Autodesk Inventor part; units mm, degrees
(part 2 of 2)
  line L144 (10.3485, -202.6701) -> (10.3485, -202.018)
  spline S172 degree 2 poles (10.3485, -202.018) (10.5375, -201.9254) (11.2155, -201.7439) (11.5193, -201.7439) knots 0 0 0 1 2 2 2
  spline S173 degree 2 poles (11.5193, -201.7439) (12.1603, -201.7439) (12.8828, -202.4219) (12.8828, -202.9999) knots 0 0 0 1 2 2 2
  spline S174 degree 2 poles (12.8828, -202.9999) (12.8828, -203.2703) (12.7568, -203.7224) (12.6456, -203.915) knots 0 0 0 1 2 2 2
  spline S175 degree 2 poles (12.6456, -203.915) (12.5345, -204.1151) (12.2122, -204.5078) (12.0343, -204.6968) knots 0 0 0 1 2 2 2
  spline S176 degree 2 poles (12.0343, -204.6968) (11.7453, -205.0117) (11.0377, -205.686) (10.8265, -205.8824) knots 0 0 0 1 2 2 2
  line L145 (10.8265, -205.8824) -> (13.0717, -205.8824)
  line L146 (13.0717, -205.8824) -> (13.0717, -206.4122)
  spline S177 degree 2 poles (14.9168, -202.2737) (14.7501, -202.2737) (14.4203, -202.3552) (14.261, -202.4182) knots 0 0 0 1 2 2 2
  spline S178 degree 2 poles (14.261, -202.4182) (14.1128, -202.4812) (13.8942, -202.6146) (13.809, -202.6738) knots 0 0 0 1 2 2 2
  line L147 (13.809, -202.6738) -> (13.772, -202.6738)
  line L148 (13.772, -202.6738) -> (13.772, -202.0255)
  spline S179 degree 2 poles (13.772, -202.0255) (13.972, -201.918) (14.6575, -201.7439) (14.965, -201.7439) knots 0 0 0 1 2 2 2
  spline S180 degree 2 poles (14.965, -201.7439) (15.2762, -201.7439) (15.7393, -201.8698) (15.9283, -202.0032) knots 0 0 0 1 2 2 2
  spline S181 degree 2 poles (15.9283, -202.0032) (16.1284, -202.1477) (16.3358, -202.5664) (16.3358, -202.848) knots 0 0 0 1 2 2 2
  spline S182 degree 2 poles (16.3358, -202.848) (16.3358, -203.2259) (15.8394, -203.7965) (15.4911, -203.8706) knots 0 0 0 1 2 2 2
  line L149 (15.4911, -203.8706) -> (15.4911, -203.915)
  spline S183 degree 2 poles (15.4911, -203.915) (15.6356, -203.9447) (15.9653, -204.078) (16.1061, -204.2114) knots 0 0 0 1 2 2 2
  spline S184 degree 2 poles (16.1061, -204.2114) (16.2469, -204.3411) (16.4248, -204.7561) (16.4248, -205.0562) knots 0 0 0 1 2 2 2
  spline S185 degree 2 poles (16.4248, -205.0562) (16.4248, -205.3637) (16.2136, -205.8861) (16.0209, -206.0862) knots 0 0 0 1 2 2 2
  spline S186 degree 2 poles (16.0209, -206.0862) (15.8208, -206.2936) (15.254, -206.5085) (14.8946, -206.5085) knots 0 0 0 1 2 2 2
  spline S187 degree 2 poles (14.8946, -206.5085) (14.55, -206.5085) (13.8757, -206.3418) (13.646, -206.227) knots 0 0 0 1 2 2 2
  line L150 (13.646, -206.227) -> (13.646, -205.5786)
  line L151 (13.646, -205.5786) -> (13.6905, -205.5786)
  spline S188 degree 2 poles (13.6905, -205.5786) (13.8831, -205.7194) (14.5352, -205.9787) (14.8575, -205.9787) knots 0 0 0 1 2 2 2
  spline S189 degree 2 poles (14.8575, -205.9787) (15.0465, -205.9787) (15.4244, -205.8602) (15.5504, -205.7231) knots 0 0 0 1 2 2 2
  spline S190 degree 2 poles (15.5504, -205.7231) (15.6726, -205.586) (15.8023, -205.2599) (15.8023, -205.0117) knots 0 0 0 1 2 2 2
  spline S191 degree 2 poles (15.8023, -205.0117) (15.8023, -204.7635) (15.6578, -204.4411) (15.5282, -204.3485) knots 0 0 0 1 2 2 2
  spline S192 degree 2 poles (15.5282, -204.3485) (15.3985, -204.2559) (15.0465, -204.1855) (14.839, -204.1855) knots 0 0 0 1 2 2 2
  line L152 (14.839, -204.1855) -> (14.5797, -204.1855)
  line L153 (14.5797, -204.1855) -> (14.5797, -203.6779)
  line L154 (14.5797, -203.6779) -> (14.7834, -203.6779)
  spline S193 degree 2 poles (14.7834, -203.6779) (15.1947, -203.6779) (15.7134, -203.2852) (15.7134, -202.911) knots 0 0 0 1 2 2 2
  spline S194 degree 2 poles (15.7134, -202.911) (15.7134, -202.7368) (15.58, -202.4886) (15.4726, -202.4145) knots 0 0 0 1 2 2 2
  spline S195 degree 2 poles (15.4726, -202.4145) (15.3577, -202.3367) (15.0761, -202.2737) (14.9168, -202.2737) knots 0 0 0 1 2 2 2
  line L155 (19.0146, -201.6364) -> (17.2251, -207.4052)
  line L156 (17.2251, -207.4052) -> (16.7063, -207.4052)
  line L157 (16.7063, -207.4052) -> (18.4885, -201.6364)
  line L158 (18.4885, -201.6364) -> (19.0146, -201.6364)
  line L159 (22.338, -206.4122) -> (19.5185, -206.4122)
  line L160 (19.5185, -206.4122) -> (19.5185, -205.7638)
  spline S196 degree 2 poles (19.5185, -205.7638) (19.8223, -205.4785) (20.3632, -204.9487) (20.6226, -204.6634) knots 0 0 0 1 2 2 2
  spline S197 degree 2 poles (20.6226, -204.6634) (21.145, -204.0892) (21.5266, -203.4) (21.5266, -203.0332) knots 0 0 0 1 2 2 2
  spline S198 degree 2 poles (21.5266, -203.0332) (21.5266, -202.8406) (21.408, -202.5516) (21.3006, -202.4589) knots 0 0 0 1 2 2 2
  spline S199 degree 2 poles (21.3006, -202.4589) (21.1931, -202.3663) (20.9116, -202.2737) (20.7411, -202.2737) knots 0 0 0 1 2 2 2
  spline S200 degree 2 poles (20.7411, -202.2737) (20.5781, -202.2737) (20.2446, -202.3552) (20.0927, -202.4182) knots 0 0 0 1 2 2 2
  spline S201 degree 2 poles (20.0927, -202.4182) (19.9631, -202.4701) (19.7222, -202.6183) (19.6481, -202.6701) knots 0 0 0 1 2 2 2
  line L161 (19.6481, -202.6701) -> (19.6148, -202.6701)
  line L162 (19.6148, -202.6701) -> (19.6148, -202.018)
  spline S202 degree 2 poles (19.6148, -202.018) (19.8037, -201.9254) (20.4818, -201.7439) (20.7856, -201.7439) knots 0 0 0 1 2 2 2
  spline S203 degree 2 poles (20.7856, -201.7439) (21.4266, -201.7439) (22.149, -202.4219) (22.149, -202.9999) knots 0 0 0 1 2 2 2
  spline S204 degree 2 poles (22.149, -202.9999) (22.149, -203.2703) (22.0231, -203.7224) (21.9119, -203.915) knots 0 0 0 1 2 2 2
  spline S205 degree 2 poles (21.9119, -203.915) (21.8008, -204.1151) (21.4784, -204.5078) (21.3006, -204.6968) knots 0 0 0 1 2 2 2
  spline S206 degree 2 poles (21.3006, -204.6968) (21.0116, -205.0117) (20.3039, -205.686) (20.0927, -205.8824) knots 0 0 0 1 2 2 2
  line L163 (20.0927, -205.8824) -> (22.338, -205.8824)
  line L164 (22.338, -205.8824) -> (22.338, -206.4122)
  spline S207 degree 2 poles (25.7948, -204.1262) (25.7948, -205.3563) (25.0797, -206.5085) (24.335, -206.5085) knots 0 0 0 1 2 2 2
  spline S208 degree 2 poles (24.335, -206.5085) (23.5792, -206.5085) (22.8715, -205.334) (22.8715, -204.1299) knots 0 0 0 1 2 2 2
  spline S209 degree 2 poles (22.8715, -204.1299) (22.8715, -202.8924) (23.5866, -201.7476) (24.335, -201.7476) knots 0 0 0 1 2 2 2
  spline S210 degree 2 poles (24.335, -201.7476) (25.0871, -201.7476) (25.7948, -202.9332) (25.7948, -204.1262) knots 0 0 0 1 2 2 2
  spline S211 degree 2 poles (25.0093, -205.5193) (25.0982, -205.2933) (25.1723, -204.5967) (25.1723, -204.1262) knots 0 0 0 1 2 2 2
  spline S212 degree 2 poles (25.1723, -204.1262) (25.1723, -203.6557) (25.0982, -202.9628) (25.0056, -202.7294) knots 0 0 0 1 2 2 2
  spline S213 degree 2 poles (25.0056, -202.7294) (24.913, -202.496) (24.5906, -202.2552) (24.335, -202.2552) knots 0 0 0 1 2 2 2
  spline S214 degree 2 poles (24.335, -202.2552) (24.0793, -202.2552) (23.7496, -202.496) (23.6533, -202.7368) knots 0 0 0 1 2 2 2
  spline S215 degree 2 poles (23.6533, -202.7368) (23.5606, -202.9702) (23.494, -203.6816) (23.494, -204.1299) knots 0 0 0 1 2 2 2
  spline S216 degree 2 poles (23.494, -204.1299) (23.494, -204.6116) (23.5532, -205.2562) (23.6496, -205.5082) knots 0 0 0 1 2 2 2
  spline S217 degree 2 poles (23.6496, -205.5082) (23.7385, -205.7453) (24.0682, -206.0009) (24.335, -206.0009) knots 0 0 0 1 2 2 2
  spline S218 degree 2 poles (24.335, -206.0009) (24.5869, -206.0009) (24.9167, -205.7601) (25.0093, -205.5193) knots 0 0 0 1 2 2 2
  line L165 (29.1997, -206.4122) -> (26.3802, -206.4122)
  line L166 (26.3802, -206.4122) -> (26.3802, -205.7638)
  spline S219 degree 2 poles (26.3802, -205.7638) (26.684, -205.4785) (27.2249, -204.9487) (27.4843, -204.6634) knots 0 0 0 1 2 2 2
  spline S220 degree 2 poles (27.4843, -204.6634) (28.0067, -204.0892) (28.3883, -203.4) (28.3883, -203.0332) knots 0 0 0 1 2 2 2
  spline S221 degree 2 poles (28.3883, -203.0332) (28.3883, -202.8406) (28.2697, -202.5516) (28.1623, -202.4589) knots 0 0 0 1 2 2 2
  spline S222 degree 2 poles (28.1623, -202.4589) (28.0548, -202.3663) (27.7733, -202.2737) (27.6028, -202.2737) knots 0 0 0 1 2 2 2
  spline S223 degree 2 poles (27.6028, -202.2737) (27.4398, -202.2737) (27.1064, -202.3552) (26.9544, -202.4182) knots 0 0 0 1 2 2 2
  spline S224 degree 2 poles (26.9544, -202.4182) (26.8248, -202.4701) (26.5839, -202.6183) (26.5098, -202.6701) knots 0 0 0 1 2 2 2
  line L167 (26.5098, -202.6701) -> (26.4765, -202.6701)
  line L168 (26.4765, -202.6701) -> (26.4765, -202.018)
  spline S225 degree 2 poles (26.4765, -202.018) (26.6655, -201.9254) (27.3435, -201.7439) (27.6473, -201.7439) knots 0 0 0 1 2 2 2
  spline S226 degree 2 poles (27.6473, -201.7439) (28.2883, -201.7439) (29.0107, -202.4219) (29.0107, -202.9999) knots 0 0 0 1 2 2 2
  spline S227 degree 2 poles (29.0107, -202.9999) (29.0107, -203.2703) (28.8848, -203.7224) (28.7736, -203.915) knots 0 0 0 1 2 2 2
  spline S228 degree 2 poles (28.7736, -203.915) (28.6625, -204.1151) (28.3401, -204.5078) (28.1623, -204.6968) knots 0 0 0 1 2 2 2
  spline S229 degree 2 poles (28.1623, -204.6968) (27.8733, -205.0117) (27.1656, -205.686) (26.9544, -205.8824) knots 0 0 0 1 2 2 2
  line L169 (26.9544, -205.8824) -> (29.1997, -205.8824)
  line L170 (29.1997, -205.8824) -> (29.1997, -206.4122)
  spline S230 degree 2 poles (32.7009, -204.9302) (32.7009, -205.2822) (32.4675, -205.8787) (32.2712, -206.0788) knots 0 0 0 1 2 2 2
  spline S231 degree 2 poles (32.2712, -206.0788) (32.0674, -206.2899) (31.5561, -206.5085) (31.2486, -206.5085) knots 0 0 0 1 2 2 2
  spline S232 degree 2 poles (31.2486, -206.5085) (30.9411, -206.5085) (30.4335, -206.3011) (30.2408, -206.0936) knots 0 0 0 1 2 2 2
  spline S233 degree 2 poles (30.2408, -206.0936) (30.0037, -205.8453) (29.7369, -205.0117) (29.7369, -204.4041) knots 0 0 0 1 2 2 2
  spline S234 degree 2 poles (29.7369, -204.4041) (29.7369, -203.8076) (29.9815, -202.848) (30.2371, -202.4923) knots 0 0 0 1 2 2 2
  spline S235 degree 2 poles (30.2371, -202.4923) (30.4853, -202.144) (31.2708, -201.755) (31.7858, -201.755) knots 0 0 0 1 2 2 2
  spline S236 degree 2 poles (31.7858, -201.755) (31.9377, -201.755) (32.2045, -201.7846) (32.3045, -201.818) knots 0 0 0 1 2 2 2
  line L171 (32.3045, -201.818) -> (32.3045, -202.4071)
  line L172 (32.3045, -202.4071) -> (32.2786, -202.4071)
  spline S237 degree 2 poles (32.2786, -202.4071) (32.1934, -202.3626) (31.8821, -202.2848) (31.7043, -202.2848) knots 0 0 0 1 2 2 2
  spline S238 degree 2 poles (31.7043, -202.2848) (31.1337, -202.2848) (30.4335, -203.0555) (30.3668, -203.8113) knots 0 0 0 1 2 2 2
  spline S239 degree 2 poles (30.3668, -203.8113) (30.5854, -203.6594) (31.0448, -203.4926) (31.319, -203.4926) knots 0 0 0 1 2 2 2
  spline S240 degree 2 poles (31.319, -203.4926) (31.5857, -203.4926) (31.9859, -203.6001) (32.2045, -203.7631) knots 0 0 0 1 2 2 2
  spline S241 degree 2 poles (32.2045, -203.7631) (32.4564, -203.9521) (32.7009, -204.5375) (32.7009, -204.9302) knots 0 0 0 1 2 2 2
  spline S242 degree 2 poles (32.0785, -204.9561) (32.0785, -204.6745) (31.9303, -204.2929) (31.7673, -204.1596) knots 0 0 0 1 2 2 2
  spline S243 degree 2 poles (31.7673, -204.1596) (31.645, -204.0632) (31.3412, -204.0002) (31.1819, -204.0002) knots 0 0 0 1 2 2 2
  spline S244 degree 2 poles (31.1819, -204.0002) (30.967, -204.0002) (30.5631, -204.1299) (30.3668, -204.2522) knots 0 0 0 1 2 2 2
  spline S245 degree 2 poles (30.3668, -204.2522) (30.3631, -204.3189) (30.3557, -204.4448) (30.3557, -204.5412) knots 0 0 0 1 2 2 2
  spline S246 degree 2 poles (30.3557, -204.5412) (30.3557, -205.0154) (30.5409, -205.5971) (30.6817, -205.749) knots 0 0 0 1 2 2 2
  spline S247 degree 2 poles (30.6817, -205.749) (30.8114, -205.8935) (31.093, -206.0084) (31.2523, -206.0084) knots 0 0 0 1 2 2 2
  spline S248 degree 2 poles (31.2523, -206.0084) (31.6228, -206.0084) (32.0785, -205.4822) (32.0785, -204.9561) knots 0 0 0 1 2 2 2
  point P0 (0, 0)
  constraints: 2 other
emboss "Emboss1" sketch "Sketch14" operation cut depth 2.54 direction (-1, 0, 0)
sketch "Sketch16" plane through (5.08, 0, 0) normal (1, 0, 0) x (0, 0, -1)
  line L0 (-45.5467, -73.9362) -> (38.2733, -73.9362)
  line L1 (38.2733, -73.9362) -> (38.2733, -77.7462)
  line L2 (38.2733, -77.7462) -> (-45.5467, -77.7462)
  line L3 (-45.5467, -77.7462) -> (-45.5467, -73.9362)
  line L4 (38.9083, -211.0962) -> (-46.1817, -211.0962) projected
  line L5 (42.0833, 28.0448) -> (42.0833, -207.9212) projected
  line L6 (-49.3567, -207.9212) -> (-49.3567, 28.0448) projected
  point P0 (0, 0)
  point P1 (38.9083, -223.7962)
  point P2 (42.0833, -220.6212)
  point P3 (38.2733, -75.8412)
  point P4 (-45.5467, -75.8412)
  dimension "d195" = 3.81
  dimension "d692" = 137.16
  dimension "d796" = 3.81
  dimension "d797" = 3.81
  constraints: 8 end point, 2 midpoint, 2 parallel, 1 horizontal, 1 perpendicular, 1 other
  measures "d195" distance between parallel lines of L0 L2
  measures "d796" distance from line of L5 point (38.273, -75.841)
  measures "d797" distance from line of L6 point (-45.547, -75.841)
extrude "Extrusion13" add sketch "Sketch16" along normal blind 5.08
sketch "Sketch17" plane through (24.13, 33.2264, 43.0067) normal (0, 1, 0) x (1, 0, 0)
  line L0 (-8.128, 57.15) -> (0, 57.15) projected
  line L1 (-0.0061, 57.15) -> (0.0392, 57.15)
  line L2 (0, 87.0966) -> (0, -8.3566) projected
  line L3 (0, 35.5801) -> (0, 35.5243)
  line L4 (5, -5.1816) -> (5, 83.9216) projected
  line L5 (0, 57.15) -> (5, 57.15)
  line L6 (5, 57.15) -> (5, 0)
  line L7 (5, 0) -> (0, 0)
  line L8 (0, 0) -> (0, 57.15)
  line L9 (0, 0) -> (-8.128, 0) projected
  point P0 (-24.13, 43.0067)
  point P1 (5, -23.8506)
  point P2 (5, 69.0626)
  point P3 (0, 0)
  point P4 (5, 57.15)
  point P5 (2.5, 0)
  point P6 (2.5, 57.15)
  dimension "d689" = 57.15
  dimension "d1196" = 0
  constraints: 12 end point, 4 point on line, 2 horizontal, 2 midpoint, 2 parallel, 1 perpendicular
  measures "d689" distance of point (2.5, 0) point (2.5, 57.15)
  measures "d1196" distance between parallel lines of L7 L9
extrude "Extrusion14" cut sketch "Sketch17" against normal blind 2.0066
sketch "Sketch18" plane through (0, 0, 0) normal (-1, 0, 0) x (0, 0, 1)
  arc A0 (48.3408, 33.2227) -> (51.3596, 30.2039) centre (50.6267, 32.4898) ccw projected
  circle A1 centre (50.6267, 32.4898) radius 4.5085
  arc A2 (-41.0674, 33.2227) -> (-44.0862, 30.2039) centre (-43.3533, 32.4898) ccw projected
  circle A3 centre (-43.3533, 32.4898) radius 4.5085
  arc A4 (-44.0862, -210.0804) -> (-41.0674, -213.0992) centre (-43.3533, -212.3662) ccw projected
  circle A5 centre (-43.3533, -212.3662) radius 4.5085
  arc A6 (48.3408, -213.0992) -> (51.3596, -210.0804) centre (50.6267, -212.3662) ccw projected
  circle A7 centre (50.6267, -212.3662) radius 4.5085
  point P0 (0, 0)
  point P1 (-44.0899, -210.0815)
  point P2 (-44.0899, -214.6509)
  point P3 (48.8233, -214.6509)
  point P4 (48.8233, -210.0815)
  point P5 (-41.0686, 33.2264)
  point P6 (-41.0686, -213.1028)
  dimension "d209" = 9.017
  dimension "d210" = 9.017
  dimension "d211" = 9.017
  dimension "d212" = 9.017
  constraints: 4 centre point, 4 coincident
  measures "d209" diameter of A1
  measures "d210" diameter of A3
  measures "d211" diameter of A5
  measures "d212" diameter of A7
extrude "Extrusion15" [suppressed]
sketch "Sketch19" plane through (24.13, -51.5842, -44.0899) normal (0, 0, -1) x (-1, 0, 0)
  line L0 (7.62, 0) -> (0, 0) projected
  line L1 (-5, 79.629) -> (-5, -156.337) projected
  line L2 (0, 0) -> (-5, 0)
  line L3 (-5, 0) -> (-5, 8.001)
  line L4 (-5, 8.001) -> (0, 8.001)
  line L5 (0, 8.001) -> (0, 0)
  point P0 (24.13, 51.5842)
  point P1 (-5, -156.337)
  dimension "d216" = 5
  dimension "d219" = 8.001
  constraints: 8 end point, 2 parallel, 1 horizontal, 1 perpendicular, 1 point on line
  measures "d216" distance between parallel lines of L1 L5
  measures "d219" distance between parallel lines of L2 L4
extrude "Extrusion16" cut sketch "Sketch19" against normal blind 24.13
sketch "Sketch20" plane through (0, 0, 0) normal (-1, 0, 0) x (0, 0, 1)
  line L0 (-45.1249, 28.9592) -> (-41.5943, 28.9592)
  line L1 (-45.1249, 36.0204) -> (-41.5943, 36.0204)
  line L2 (-45.1249, 28.9592) -> (-47.1633, 32.4898)
  line L3 (-45.1249, 36.0204) -> (-47.1633, 32.4898)
  line L4 (-41.5943, 28.9592) -> (-39.5559, 32.4898)
  line L5 (-41.5943, 36.0204) -> (-39.5559, 32.4898)
  line L6 (-45.1249, -215.8968) -> (-41.5943, -215.8968)
  line L7 (-45.1249, -208.8356) -> (-41.5943, -208.8356)
  line L8 (-45.1249, -215.8968) -> (-47.1633, -212.3662)
  line L9 (-45.1249, -208.8356) -> (-47.1633, -212.3662)
  line L10 (-41.5943, -215.8968) -> (-39.5559, -212.3662)
  line L11 (-41.5943, -208.8356) -> (-39.5559, -212.3662)
  line L12 (48.8551, 28.9592) -> (52.3857, 28.9592)
  line L13 (48.8551, 36.0204) -> (52.3857, 36.0204)
  line L14 (48.8551, 28.9592) -> (46.8167, 32.4898)
  line L15 (48.8551, 36.0204) -> (46.8167, 32.4898)
  line L16 (52.3857, 28.9592) -> (54.4241, 32.4898)
  line L17 (52.3857, 36.0204) -> (54.4241, 32.4898)
  line L18 (48.8551, -215.8968) -> (52.3857, -215.8968)
  line L19 (48.8551, -208.8356) -> (52.3857, -208.8356)
  line L20 (48.8551, -215.8968) -> (46.8167, -212.3662)
  line L21 (48.8551, -208.8356) -> (46.8167, -212.3662)
  line L22 (52.3857, -215.8968) -> (54.4241, -212.3662)
  line L23 (52.3857, -208.8356) -> (54.4241, -212.3662)
  line L24 (-40.0449, -67.5608) -> (-36.5143, -67.5608)
  line L25 (-40.0449, -60.4996) -> (-36.5143, -60.4996)
  line L26 (-40.0449, -67.5608) -> (-42.0833, -64.0302)
  line L27 (-40.0449, -60.4996) -> (-42.0833, -64.0302)
  line L28 (-36.5143, -67.5608) -> (-34.4759, -64.0302)
  line L29 (-36.5143, -60.4996) -> (-34.4759, -64.0302)
  line L30 (43.7751, -67.5608) -> (47.3057, -67.5608)
  line L31 (43.7751, -60.4996) -> (47.3057, -60.4996)
  line L32 (43.7751, -67.5608) -> (41.7367, -64.0302)
  line L33 (43.7751, -60.4996) -> (41.7367, -64.0302)
  line L34 (47.3057, -67.5608) -> (49.3441, -64.0302)
  line L35 (47.3057, -60.4996) -> (49.3441, -64.0302)
  point P0 (0, 0)
  point P1 (-16.6833, 31.2198)
  point P2 (-43.3596, 28.9592)
  point P3 (-43.3533, 32.4898)
  point P4 (-43.3596, -215.8968)
  point P5 (50.6204, 28.9592)
  point P6 (50.6204, -215.8968)
  point P7 (-38.2796, -67.5608)
  point P8 (45.5404, -67.5608)
  dimension "d963" = 7.0612
  dimension "d964" = 120
  dimension "d965" = 120
  dimension "d966" = 120
  dimension "d967" = 120
  dimension "d968" = 3.5306
  dimension "d969" = 3.5306
  dimension "d970" = 3.5306
  dimension "d971" = 3.5306
  dimension "d972" = 3.5306
  dimension "d973" = 3.5306
  dimension "d974" = 0
  dimension "d975" = 7.6074
  dimension "d1031" = 7.0612
  dimension "d1032" = 120
  dimension "d1033" = 120
  dimension "d1034" = 120
  dimension "d1035" = 120
  dimension "d1036" = 3.5306
  dimension "d1037" = 3.5306
  dimension "d1038" = 3.5306
  dimension "d1039" = 3.5306
  dimension "d1040" = 3.5306
  dimension "d1041" = 3.5306
  dimension "d1042" = 0
  dimension "d1043" = 7.6074
  dimension "d1082" = 7.0612
  dimension "d1083" = 120
  dimension "d1084" = 120
  dimension "d1085" = 120
  dimension "d1086" = 120
  dimension "d1087" = 3.5306
  dimension "d1088" = 3.5306
  dimension "d1089" = 3.5306
  dimension "d1090" = 3.5306
  dimension "d1091" = 3.5306
  dimension "d1092" = 3.5306
  dimension "d1093" = 0
  dimension "d1094" = 7.6074
  dimension "d1116" = 7.0612
  dimension "d1117" = 120
  dimension "d1118" = 120
  dimension "d1119" = 120
  dimension "d1120" = 120
  dimension "d1121" = 3.5306
  dimension "d1122" = 3.5306
  dimension "d1123" = 3.5306
  dimension "d1124" = 3.5306
  dimension "d1125" = 3.5306
  dimension "d1126" = 3.5306
  dimension "d1127" = 0
  dimension "d1128" = 7.6074
  dimension "d1160" = 7.0612
  dimension "d1161" = 120
  dimension "d1162" = 120
  dimension "d1163" = 120
  dimension "d1164" = 120
  dimension "d1165" = 3.5306
  dimension "d1166" = 3.5306
  dimension "d1167" = 3.5306
  dimension "d1168" = 3.5306
  dimension "d1169" = 3.5306
  dimension "d1170" = 3.5306
  dimension "d1171" = 0
  constraints: 72 end point, 12 horizontal, 6 midpoint
  measures "d963" distance from line of point (-43.36, 28.959) L1
  measures "d964" angle of L0 L2
  measures "d965" angle of L1 L3
  measures "d966" angle of L4 L0
  measures "d967" angle of L5 L1
  measures "d968" distance of L0.start L4.start
  measures "d969" distance of L1.start L5.start
  measures "d970" vertical distance of L1.start L3.end
  measures "d971" vertical distance of L0.start L2.end
  measures "d972" vertical distance of L5.start L5.end
  measures "d973" vertical distance of L4.start L4.end
  measures "d974" horizontal distance of L0.start L1.start
  measures "d975" distance of L4.end L2.end
  measures "d1031" distance from line of point (-43.36, -215.897) L7
  measures "d1032" angle of L6 L8
  measures "d1033" angle of L7 L9
  measures "d1034" angle of L10 L6
  measures "d1035" angle of L11 L7
  measures "d1036" distance of L6.start L10.start
  measures "d1037" distance of L7.start L11.start
  measures "d1038" vertical distance of L7.start L9.end
  measures "d1039" vertical distance of L6.start L8.end
  measures "d1040" vertical distance of L11.start L11.end
  measures "d1041" vertical distance of L10.start L10.end
  measures "d1042" horizontal distance of L6.start L7.start
  measures "d1043" distance of L10.end L8.end
  measures "d1082" distance from line of point (50.62, 28.959) L13
  measures "d1083" angle of L12 L14
  measures "d1084" angle of L13 L15
  measures "d1085" angle of L16 L12
  measures "d1086" angle of L17 L13
  measures "d1087" distance of L12.start L16.start
  measures "d1088" distance of L15.start L17.start
  measures "d1089" vertical distance of L15.start L15.end
  measures "d1090" vertical distance of L12.start L14.end
  measures "d1091" vertical distance of L17.start L17.end
  measures "d1092" vertical distance of L16.start L16.end
  measures "d1093" horizontal distance of L12.start L15.start
  measures "d1094" distance of L16.end L14.end
  measures "d1116" distance from line of point (50.62, -215.897) L19
  measures "d1117" angle of L18 L20
  measures "d1118" angle of L19 L21
  measures "d1119" angle of L22 L18
  measures "d1120" angle of L23 L19
  measures "d1121" distance of L18.start L22.start
  measures "d1122" distance of L21.start L23.start
  measures "d1123" vertical distance of L21.start L21.end
  measures "d1124" vertical distance of L18.start L20.end
  measures "d1125" vertical distance of L23.start L23.end
  measures "d1126" vertical distance of L22.start L22.end
  measures "d1127" horizontal distance of L18.start L21.start
  measures "d1128" distance of L22.end L20.end
  measures "d1160" distance from line of point (-38.28, -67.561) L25
  measures "d1161" angle of L24 L26
  measures "d1162" angle of L25 L27
  measures "d1163" angle of L28 L24
  measures "d1164" angle of L29 L25
  measures "d1165" distance of L24.start L28.start
  measures "d1166" distance of L25.start L29.start
  measures "d1167" vertical distance of L25.start L27.end
  measures "d1168" vertical distance of L24.start L26.end
  measures "d1169" vertical distance of L29.start L29.end
  measures "d1170" vertical distance of L28.start L28.end
  measures "d1171" horizontal distance of L24.start L25.start
extrude "Extrusion18" cut sketch "Sketch20" against normal blind 4
sketch "Sketch21" plane through (5.08, 0, 0) normal (1, 0, 0) x (0, 0, -1)
  line L0 (-49.3567, -207.9212) -> (-49.3567, 28.0448) projected
  line L1 (42.0833, -69.6717) -> (42.0833, -83.8957)
  line L2 (44.0899, -209.9278) -> (44.0899, -51.5842) projected
  line L3 (-49.3567, -83.8422) -> (-49.3567, -69.6182)
  line L4 (-42.4987, -58.8939) -> (-42.4987, -69.23)
  line L5 (-44.2301, -72.0578) -> (-47.3797, -73.6657)
  line L6 (-48.7308, -74.9867) -> (-49.3567, -76.1476)
  line L7 (-44.2301, -56.0661) -> (-47.3797, -54.4582)
  line L8 (-48.7639, -53.074) -> (-49.3567, -51.9128)
  arc A0 (-47.3797, -73.6657) -> (-48.7308, -74.9867) centre (-45.9361, -76.4935) ccw
  arc A1 (-44.2301, -72.0578) -> (-42.4987, -69.23) centre (-45.6737, -69.23) ccw
  arc A2 (-42.4987, -58.8939) -> (-44.2301, -56.0661) centre (-45.6737, -58.8939) ccw
  arc A3 (-48.7639, -53.074) -> (-47.3797, -54.4582) centre (-45.9361, -51.6304) ccw
  line L9 (-49.3567, -51.9128) -> (-49.3567, -76.1476)
  arc A4 (-47.9472, -64.0302) -> (-47.9472, -64.0302) centre (-45.5467, -64.0302) ccw projected
  circle A5 centre (-45.5467, -64.0302) radius 2.4005
  line L10 (35.2253, -69.1835) -> (35.2253, -58.8478)
  line L11 (36.9569, -56.0198) -> (40.1065, -54.4123)
  line L12 (41.4675, -53.0729) -> (42.0833, -51.9128)
  line L13 (36.9569, -72.0115) -> (40.1065, -73.619)
  line L14 (41.4675, -74.9584) -> (42.0833, -76.1184)
  arc A6 (41.4675, -74.9584) -> (40.1065, -73.619) centre (38.6631, -76.447) ccw
  arc A7 (35.2253, -69.1835) -> (36.9569, -72.0115) centre (38.4003, -69.1835) ccw
  arc A8 (40.1065, -54.4123) -> (41.4675, -53.0729) centre (38.6631, -51.5843) ccw
  arc A9 (36.9569, -56.0198) -> (35.2253, -58.8478) centre (38.4003, -58.8478) ccw
  line L15 (42.0833, -51.9128) -> (42.0833, -76.1184)
  line L16 (42.0833, -51.9128) -> (42.0833, -76.1184)
  circle A10 centre (38.2733, -64.0302) radius 2.4005 projected
  line L17 (42.0833, -51.5842) -> (42.0833, -43.5842) projected
  circle A11 centre (53.1966, -64.0156) radius 2.0413
  point P0 (0, 0)
  point P1 (-43.0067, -58.9502)
  point P2 (-48.2611, -74.1156)
  point P3 (-48.2961, -53.9904)
  point P4 (-43.0067, -74.3297)
  point P5 (-40.8318, -77.7462)
  point P6 (40.9982, -53.9572)
  dimension "d785" = 6.858
  dimension "d786" = 117.044
  dimension "d787" = 117.044
  dimension "d792" = 2.032
  dimension "d793" = 3.175
  dimension "d794" = 3.1496
  dimension "d795" = 3.1496
  dimension "d917" = 24.2348
  dimension "d1137" = 4.801
  dimension "d1144" = 145
  dimension "d1145" = 145
  dimension "d1146" = 117.04
  dimension "d1147" = 117.04
  dimension "d1148" = 3.175
  dimension "d1149" = 3.175
  dimension "d1150" = 3.1496
  dimension "d1151" = 2.0443
  dimension "d1152" = 3.1496
  dimension "d1153" = 24.2056
  dimension "d1155" = 0
  dimension "d1156" = 12.1028
  dimension "d1157" = 14.9233
  dimension "d1158" = 12.1174
  dimension "d1159" = 12.1174
  constraints: 30 end point, 16 point on circle, 16 tangent, 10 centre point, 9 point on line, 5 equal radius, 2 vertical, 1 coincident, 1 collinear, 1 parallel, 1 perpendicular
  measures "d785" distance between parallel lines of L0 L4
  measures "d786" angle of L5 L4
  measures "d787" angle of L7 L4
  measures "d792" vertical distance of point (-48.261, -74.116) L6.end
  measures "d793" radius of A0
  measures "d794" horizontal distance of L5.start L5.end
  measures "d795" horizontal distance of L7.start L7.end
  measures "d917" distance of L6.end L8.end
  measures "d1137" diameter of A5
  measures "d1144" angle of L11 L12
  measures "d1145" angle of L14 L13
  measures "d1146" angle of L13 L10
  measures "d1147" angle of L10 L11
  measures "d1148" radius of A6
  measures "d1149" radius of A8
  measures "d1150" horizontal distance of L11.start L11.end
  measures "d1151" vertical distance of L12.end point (40.998, -53.957)
  measures "d1152" horizontal distance of L13.start L13.end
  measures "d1153" distance of L14.end L12.end
  measures "d1155" distance between parallel lines of L17 L15
  measures "d1156" vertical distance of L12.end A11.centre
  measures "d1157" distance of A10.centre A11.centre
  measures "d1158" vertical distance of A4.centre L8.end
  measures "d1159" vertical distance of A10.centre L12.end
extrude "Extrusion19" add sketch "Sketch21" along normal blind 22.86 contours L0 L8 A3 L7 A2 L4 A1 L5 A0 L6 | L1 L14 A6 L13 A7 L10 A9 L11 A8 L12 L15
sketch "Sketch22" plane through (16.08, -230.1462, -3.2973) normal (0, -1, 0) x (1, 0, 0)
  circle A0 centre (2.2292, -12.1283) radius 2.032
  line L0 (-16.08, -45.136) -> (8.05, -45.136) projected
  circle A1 centre (10.002, -12.1283) radius 2.032
  line L1 (13.05, 48.9456) -> (13.05, -37.6176) projected
  point P0 (-16.08, 3.2973)
  dimension "d445" = 4.064
  dimension "d446" = 33.0076
  dimension "d449" = 4.064
  dimension "d450" = 3.048
  constraints: 2 centre point
  measures "d445" diameter of A0
  measures "d446" distance from line of L0 A0.centre
  measures "d449" diameter of A1
  measures "d450" distance from line of L1 A1.centre
extrude "Extrusion20" [suppressed]
fillet "Fillet6" radius 0.508 8 edges at (20.32, -51.5842, -48.4333) (20.32, -43.5842, -48.4333) (16.51, -47.5842, -48.4333) (20.066, 37.5698, -14.1433) (16.002, 37.5698, 14.4317) (20.066, 37.5698, 43.0067) (26.63, 33.2264, 43.0067) (26.63, -43.5832, -44.0899)
sketch "Sketch23" plane through (22.86, -225.8028, -3.2973) normal (0, -1, 0) x (1, 0, 0)
  line L0 (1.27, -37.6176) -> (1.27, 48.9456) projected
  line L1 (6.27, 48.9456) -> (6.27, -37.6176) projected
  line L2 (0, 10) -> (6.27, 10)
  line L3 (6.27, 10) -> (6.27, -0.0129)
  line L4 (6.27, -0.0129) -> (0, -0.0129)
  line L5 (0, -0.0129) -> (0, 10)
  point P0 (-22.86, 3.2973)
  point P1 (1.27, 48.9456)
  constraints: 8 end point, 2 parallel, 1 horizontal, 1 perpendicular, 1 point on line, 1 other
extrude "Extrusion21" [suppressed]
sketch "Sketch24" plane through (8.636, -223.7962, -3.2973) normal (0, 1, 0) x (1, 0, 0)
  circle A0 centre (9.652, -31.318) radius 4.445
  line L0 (-3.556, 35.611) -> (-3.556, -46.939) projected
  point P0 (-8.636, -3.2973)
  point P1 (15.494, -56.464)
  dimension "d673" = 25.146
  dimension "d674" = 13.208
  dimension "d677" = 8.89
  constraints: 1 centre point
  measures "d673" vertical distance of point (15.494, -56.464) A0.centre
  measures "d674" distance from line of L0 A0.centre
  measures "d677" diameter of A0
extrude "Extrusion22" [suppressed]
sketch "Sketch25" plane through (5.08, 0, 0) normal (1, 0, 0) x (0, 0, -1)
  line L0 (-49.3567, 15.9798) -> (20.6609, 15.9798)
  line L1 (11.7709, 3.2798) -> (-49.3567, 3.2798)
  line L2 (-49.3567, 3.2798) -> (-49.3567, 15.9798)
  circle A0 centre (-32.8467, 9.6298) radius 2.4005 projected
  circle A1 centre (4.1509, 9.6298) radius 2.4005 projected
  circle A2 centre (-14.3479, 9.6298) radius 2.4005 projected
  line L3 (-49.3567, -207.9212) -> (-49.3567, 28.0448) projected
  line L4 (42.0833, 28.0448) -> (42.0833, -43.5832) projected
  line L5 (20.6609, 15.9798) -> (42.0833, 15.9798)
  line L6 (42.0833, 15.9798) -> (42.0833, 3.2798)
  line L7 (42.0833, 3.2798) -> (11.7709, 3.2798)
  point P0 (0, 0)
  point P1 (-14.3479, 15.9798)
  point P2 (-46.8167, -36.8286)
  point P3 (-49.3567, 28.0448)
  point P4 (42.0833, -36.6918)
  dimension "d680" = 6.35
  dimension "d681" = 6.35
  dimension "d682" = 0
  dimension "d685" = 0
  dimension "d686" = 12.7
  constraints: 12 end point, 2 horizontal, 2 parallel, 1 midpoint, 1 perpendicular, 1 other
  measures "d680" distance of point (-14.348, 15.98) A2.centre
  measures "d681" distance from line of L1 A2.centre
  measures "d682" horizontal extent of L2
  measures "d685" distance between parallel lines of L4 L6
  measures "d686" distance between parallel lines of L7 L5
extrude "Extrusion23" add sketch "Sketch25" along normal blind 10.16
sketch "Sketch26" plane through (0, -217.4462, -45.2583) normal (0, -1, 0) x (1, 0, 0)
  line L0 (29.13, 88.265) -> (10.3097, 88.265)
  line L1 (10.3097, 9.525) -> (29.13, 9.525)
  line L2 (29.13, 9.525) -> (29.13, 88.265)
  line L3 (0, -3.175) -> (24.13, -3.175) projected
  line L4 (24.13, 100.965) -> (0, 100.965) projected
  line L5 (29.13, 93.4466) -> (29.13, 4.3434) projected
  line L6 (8.7811, 88.265) -> (8.7811, 85.0428)
  line L7 (10.3097, 88.265) -> (8.7811, 88.265)
  line L8 (8.7811, 88.265) -> (8.7811, 9.525)
  line L9 (10.3097, 9.525) -> (8.7811, 9.525)
  point P0 (0, 45.2583)
  point P1 (29.13, 51.961)
  dimension "d832" = 12.7
  dimension "d833" = 12.7
  dimension "d837" = 0
  constraints: 14 end point, 2 horizontal, 2 perpendicular, 1 parallel, 1 vertical
  measures "d832" distance between parallel lines of L3 L1
  measures "d833" distance between parallel lines of L4 L0
  measures "d837" distance between parallel lines of L5 L2
extrude "Extrusion24" cut sketch "Sketch26" against normal blind 7.62
fillet "Fillet7" radius 0.762 4 edges at (17.2199, -217.4462, 43.0067) (9.5454, -217.4462, 43.0067) (17.2199, -217.4462, -35.7333) (9.5454, -217.4462, -35.7333)
body "Solid1"
